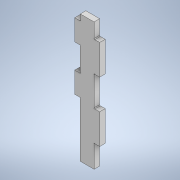
# Autodesk Inventor part: cover
Saved by Autodesk Inventor 2020 (Build 240168000, 168)
## iProperties
Created: 2019-12-19
Part Number: cover
Material: Générique
Document SubType Name: Modeling
Designer: damien
Density: 1 g/cm^3
Appearance: Par défaut
Author: damien
Autodesk Inventor part; units mm, degrees
ref_plane "YZ Plane" through (0, 0, 0) normal (1, 0, 0) x (0, 1, 0)
ref_plane "XZ Plane" through (0, 0, 0) normal (0, 1, 0) x (-1, 0, 0)
ref_plane "XY Plane" through (0, 0, 0) normal (0, 0, 1) x (1, 0, 0)
sketch "Esquisse3" plane through (0, 0, 0) normal (0, 0, 1) x (1, 0, 0)
  line L0 (41.5, -212.5) -> (-41.5, -212.5)
  line L1 (-41.5, -212.5) -> (-41.5, 212.5)
  line L2 (-41.5, 212.5) -> (41.5, 212.5)
  line L3 (41.5, 212.5) -> (41.5, -212.5)
  line L4 (41.5, -212.5) -> (-41.5, 212.5) construction
  line L5 (-41.5, -212.5) -> (41.5, 212.5) construction
  point P0 (0, 0)
  dimension "d20" = 83
  dimension "d21" = 425
  constraints: 12 end point, 2 midpoint, 2 parallel, 1 horizontal, 1 perpendicular
  measures "d20" distance of L0.start L0.end
  measures "d21" distance of L2.end L0.start
extrude "Extrusion3" add sketch "Esquisse3" along normal blind 18.55
sketch "Esquisse4" plane through (0, 0, 18.55) normal (0, 0, 1) x (1, 0, 0)
  line L0 (41.5, 212.5) -> (22.9, 212.5)
  line L1 (22.9, 212.5) -> (22.9, 162.5)
  line L2 (22.9, 162.5) -> (41.5, 162.5)
  line L3 (41.5, 162.5) -> (41.5, 212.5)
  line L4 (-41.5, -212.5) -> (41.5, -212.5) projected
  line L5 (41.5, -212.5) -> (22.9, -212.5)
  line L6 (22.9, -212.5) -> (22.9, -137.5)
  line L7 (22.9, -137.5) -> (41.5, -137.5)
  line L8 (41.5, -137.5) -> (41.5, -212.5)
  line L9 (41.5, -37.5) -> (22.9, -37.5)
  line L10 (22.9, -37.5) -> (22.9, 62.5)
  line L11 (22.9, 62.5) -> (41.5, 62.5)
  line L12 (41.5, 62.5) -> (41.5, -37.5)
  point P0 (0, 0)
  dimension "d24" = 75
  dimension "d25" = 50
  dimension "d27" = 100
  dimension "d29" = 100
  dimension "d30" = 100
  dimension "d31" = 18.6
  constraints: 24 end point, 6 parallel, 3 horizontal, 3 perpendicular, 2 collinear, 1 point on line
  measures "d24" distance of L5.end L6.end
  measures "d25" distance of L0.end L1.end
  measures "d27" distance of L9.end L10.end
  measures "d29" distance between parallel lines of L7 L9
  measures "d30" distance between parallel lines of L2 L11
  measures "d31" distance between parallel lines of L12 L10
extrude "Extrusion4" cut sketch "Esquisse4" against normal blind 18.55
sketch "Esquisse5" plane through (0, 0, 18.55) normal (0, 0, 1) x (1, 0, 0)
  line L0 (22.9, 212.5) -> (-41.5, 212.5) projected
  line L1 (-41.5, 212.5) -> (-22.95, 212.5)
  line L2 (-22.95, 212.5) -> (-22.95, 192.5)
  line L3 (-22.95, 192.5) -> (-41.5, 192.5)
  line L4 (-41.5, 192.5) -> (-41.5, 212.5)
  line L5 (-41.5, 212.5) -> (-41.5, -212.5) projected
  line L6 (-41.5, 122.5) -> (-22.95, 122.5)
  line L7 (-22.95, 122.5) -> (-22.95, 41.5)
  line L8 (-22.95, 41.5) -> (-41.5, 41.5)
  line L9 (-41.5, 41.5) -> (-41.5, 122.5)
  line L10 (-41.5, -28.5) -> (-22.95, -28.5)
  line L11 (-22.95, -28.5) -> (-22.95, -212.5)
  line L12 (-22.95, -212.5) -> (-41.5, -212.5)
  line L13 (-41.5, -212.5) -> (-41.5, -28.5)
  line L14 (-41.5, -212.5) -> (22.9, -212.5) projected
  point P0 (0, 0)
  point P1 (-41.5, 41.5)
  dimension "d34" = 20
  dimension "d35" = 18.55
  dimension "d37" = 70
  dimension "d38" = 81
  dimension "d39" = 70
  constraints: 24 end point, 6 parallel, 3 collinear, 3 horizontal, 3 perpendicular, 2 point on line
  measures "d34" distance of L3.end L0.end
  measures "d35" distance from line of L2 L3.end
  measures "d37" distance between parallel lines of L6 L3
  measures "d38" distance of L6.end L7.end
  measures "d39" distance between parallel lines of L10 L8
extrude "Extrusion5" cut sketch "Esquisse5" against normal blind 18.55
sketch "Esquisse6" plane through (0, 0, 18.55) normal (0, 0, 1) x (1, 0, 0)
  circle A0 centre (-24.0708, 193.6208) radius 1.585
  circle A1 centre (24.0208, 163.6208) radius 1.585
  circle A2 centre (-24.0708, 121.3792) radius 1.585
  circle A3 centre (24.0208, 61.3792) radius 1.585
  circle A4 centre (-24.0708, 42.6208) radius 1.585
  circle A5 centre (24.0208, -36.3792) radius 1.585
  circle A6 centre (-24.0708, -29.6208) radius 1.585
  circle A7 centre (24.0208, -138.6208) radius 1.585
  line L0 (-41.5, 192.5) -> (-22.95, 192.5) projected
  line L1 (-24.0708, 193.6208) -> (-22.95, 192.5) construction
  line L2 (41.5, 162.5) -> (22.9, 162.5) projected
  line L3 (22.9, 162.5) -> (24.0208, 163.6208) construction
  line L4 (-22.95, 122.5) -> (-41.5, 122.5) projected
  line L5 (-22.95, 122.5) -> (-24.0708, 121.3792) construction
  line L6 (-24.0708, 42.6208) -> (-22.95, 41.5) construction
  line L7 (-41.5, 41.5) -> (-22.95, 41.5) projected
  line L8 (22.9, 62.5) -> (24.0208, 61.3792) construction
  line L9 (-22.95, -28.5) -> (-41.5, -28.5) projected
  line L10 (-22.95, -28.5) -> (-24.0708, -29.6208) construction
  line L11 (-22.95, -28.5) -> (-22.95, -212.5) projected
  line L12 (41.5, -37.5) -> (22.9, -37.5) projected
  line L13 (22.9, -37.5) -> (24.0208, -36.3792) construction
  line L14 (22.9, -37.5) -> (22.9, 62.5) projected
  line L15 (22.9, -137.5) -> (41.5, -137.5) projected
  line L16 (22.9, -137.5) -> (24.0208, -138.6208) construction
  point P0 (0, 0)
  dimension "d43" = 3.17
  dimension "d46" = 45
  dimension "d47" = 45
  dimension "d49" = 45
  dimension "d51" = 45
  dimension "d52" = 45
  dimension "d53" = 45
  dimension "d54" = 45
  constraints: 16 end point, 2 point on circle, 1 centre point, 1 point on line, 1 vertical alignment, 22 other
  measures "d46" angle of L0 L1
  measures "d47" angle of L2 L3
  measures "d49" angle of L7 L6
  measures "d51" angle of L11 L10
  measures "d52" angle of L12 L13
  measures "d53" angle of L14 L8
  measures "d54" angle of L15 L16
extrude "Extrusion6" cut sketch "Esquisse6" against normal blind 18.55
